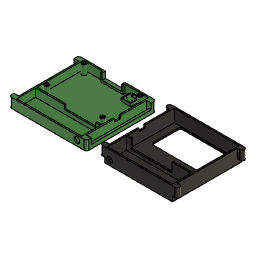
case (Autodesk Fusion 360 design; units mm, degrees)
Autodesk Fusion 360 part; units mm, degrees
(part 1 of 2)
sketch "Sketch1" plane through (0, 0, 0) normal (0, 0, 1) x (1, 0, 0)
  line L0 (0, 0) -> (127, 0)
  line L1 (127, 0) -> (127, 88)
  line L2 (127, 88) -> (0, 88)
  line L3 (0, 88) -> (0, 0)
  circle A0 centre (5, 82.8) radius 3
  circle A1 centre (121.74, 82.8) radius 3
  circle A2 centre (5, 5) radius 3
  circle A3 centre (121.74, 5) radius 3
  circle A4 centre (5, 71.19) radius 3.5
  circle A5 centre (121.74, 71.19) radius 3.5
  circle A6 centre (5, 33.49) radius 3.5
  circle A7 centre (121.74, 33.49) radius 3.5
  line L4 (8, 84.5321) -> (5, 86.2641)
  line L5 (5, 86.2641) -> (2, 84.5321)
  line L6 (2, 84.5321) -> (2, 81.0679)
  line L7 (2, 81.0679) -> (5, 79.3359)
  line L8 (5, 79.3359) -> (8, 81.0679)
  line L9 (8, 81.0679) -> (8, 84.5321)
  line L10 (123.4721, 79.8) -> (125.2041, 82.8)
  line L11 (125.2041, 82.8) -> (123.4721, 85.8)
  line L12 (123.4721, 85.8) -> (120.0079, 85.8)
  line L13 (120.0079, 85.8) -> (118.2759, 82.8)
  line L14 (118.2759, 82.8) -> (120.0079, 79.8)
  line L15 (120.0079, 79.8) -> (123.4721, 79.8)
  line L16 (123.4721, 2) -> (125.2041, 5)
  line L17 (125.2041, 5) -> (123.4721, 8)
  line L18 (123.4721, 8) -> (120.0079, 8)
  line L19 (120.0079, 8) -> (118.2759, 5)
  line L20 (118.2759, 5) -> (120.0079, 2)
  line L21 (120.0079, 2) -> (123.4721, 2)
  line L22 (8, 6.7321) -> (5, 8.4641)
  line L23 (5, 8.4641) -> (2, 6.7321)
  line L24 (2, 6.7321) -> (2, 3.2679)
  line L25 (2, 3.2679) -> (5, 1.5359)
  line L26 (5, 1.5359) -> (8, 3.2679)
  line L27 (8, 3.2679) -> (8, 6.7321)
  point P0 (5, 82.8)
  point P1 (121.74, 82.8)
  point P2 (121.74, 5)
  point P3 (5, 5)
  dimension "d1" = 127
  dimension "d2" = 88
  dimension "d3" = 6
  dimension "d4" = 6
  dimension "d5" = 6
  dimension "d6" = 6
  dimension "d7" = 5.2
  dimension "d8" = 5
  dimension "d9" = 5
  dimension "d10" = 5.26
  dimension "d11" = 7
  dimension "d12" = 7
  dimension "d13" = 7
  dimension "d14" = 7
  dimension "d15" = 11.61
  dimension "d16" = 28.49
  constraint horizontal L0
  constraint vertical L1
  constraint horizontal L2
  constraint vertical L3
  constraint coincident L0.start L3.end
  constraint vertical P0 P3
  constraint vertical P1 P2
  constraint horizontal P0 P1
  constraint horizontal P3 P2
  constraint vertical A4.centre A6.centre
  constraint vertical A5.centre A7.centre
  constraint horizontal A6.centre A7.centre
  constraint horizontal A4.centre A5.centre
  constraint vertical P0 A4.centre
  constraint vertical P1 A5.centre
  constraint coincident P0 A0.centre
  constraint coincident P1 A1.centre
  constraint coincident P2 A3.centre
  constraint coincident P3 A2.centre
  measures "d1" distance of L1.end L2.end
  measures "d2" distance of L0.end L1.end
  measures "d3" diameter of A0
  measures "d4" diameter of A1
  measures "d5" diameter of A2
  measures "d6" diameter of A3
  measures "d7" distance of L2 P0
  measures "d8" distance of L0 P3
  measures "d9" distance of L3 P0
  measures "d10" distance of L1 P1
  measures "d11" diameter of A4
  measures "d12" diameter of A5
  measures "d13" diameter of A6
  measures "d14" diameter of A7
  measures "d15" distance of P0 A4.centre
  measures "d16" distance of P3 A6.centre
extrude "Extrude1" add sketch "Sketch1" along normal blind 1.25 contours L0 L1 L2 L3 | A0 L8 L9 | A0 L4 L9 | A0 L4 L5 | A0 L7 L8 | A0 L5 L6 | A0 L6 L7 | A1 L10 L11 | A1 L11 L12 | A1 L10 L15 | A1 L12 L13 | A1 L14 L15 | A1 L13 L14 | A2 L26 L27 | A2 L22 L27 | A2 L22 L23 | A2 L25 L26 | A2 L23 L24 | A2 L24 L25 | A3 L16 L17 | A3 L17 L18 | A3 L16 L21 | A3 L18 L19 | A3 L20 L21 | A3 L19 L20 makes body 1
extrude "Extrude1'" add sketch "Sketch1" against normal blind 13 separate body contours A0 | A0 L8 L9 | A0 L4 L9 | A0 L4 L5 | A0 L7 L8 | A0 L5 L6 | A0 L6 L7 | A1 | A1 L10 L11 | A1 L11 L12 | A1 L10 L15 | A1 L12 L13 | A1 L14 L15 | A1 L13 L14 | A2 | A2 L26 L27 | A2 L22 L27 | A2 L22 L23 | A2 L25 L26 | A2 L23 L24 | A2 L24 L25 | A3 | A3 L16 L17 | A3 L17 L18 | A3 L16 L21 | A3 L18 L19 | A3 L20 L21 | A3 L19 L20 makes body 2 at (118.8532, 81.8, -4.3333) makes body 3 at (7, 85.1094, -4.3333) makes body 4 at (122.3174, 8, -4.3333) makes body 5 at (8, 4.4226, -4.3333) in component "Component"
extrude "Extrude1''" add sketch "Sketch1" along normal blind 3.25 separate body contours A0 | A1 | A2 | A3 makes body 6 at (7.7644, 81.6347, 1.0833) makes body 7 at (124.5044, 81.6347, 1.0833) makes body 8 at (7.9851, 4.7013, 1.0833) makes body 9 at (121.2191, 7.9544, 2.1667) in component "Component'"
fillet "Fillet1" radius 1 4 edges at (2.203, 81.7152, 3.25) (118.943, 81.7152, 3.25) (2.203, 3.9152, 3.25) (118.943, 3.9152, 3.25) on bodies 6 7 8 9 in component "Component'"
sketch "Sketch2" plane through (0, 0, 1.25) normal (0, 0, 1) x (-1, 0, 0)
  circle A0 centre (-121.74, -82.8) radius 3
  circle A1 centre (-121.74, -5) radius 3
  circle A2 centre (-5, -71.19) radius 3.5
  circle A3 centre (-121.74, -71.19) radius 3.5
  circle A4 centre (-5, -5) radius 3
  circle A5 centre (-5, -33.49) radius 3.5
  circle A6 centre (-121.74, -33.49) radius 3.5
  circle A7 centre (-5, -82.8) radius 3
  line L0 (0, -88) -> (0, 0)
  line L1 (0, 0) -> (-127, 0)
  line L2 (-127, 0) -> (-127, -88)
  line L3 (-127, -88) -> (0, -88)
  line L4 (-8.5, -73.2107) -> (-5, -75.2315)
  line L5 (-5, -75.2315) -> (-1.5, -73.2107)
  line L6 (-1.5, -73.2107) -> (-1.5, -69.1693)
  line L7 (-1.5, -69.1693) -> (-5, -67.1485)
  line L8 (-5, -67.1485) -> (-8.5, -69.1693)
  line L9 (-8.5, -69.1693) -> (-8.5, -73.2107)
  line L10 (-123.7607, -67.69) -> (-125.7815, -71.19)
  line L11 (-125.7815, -71.19) -> (-123.7607, -74.69)
  line L12 (-123.7607, -74.69) -> (-119.7193, -74.69)
  line L13 (-119.7193, -74.69) -> (-117.6985, -71.19)
  line L14 (-117.6985, -71.19) -> (-119.7193, -67.69)
  line L15 (-119.7193, -67.69) -> (-123.7607, -67.69)
  line L16 (-123.7607, -29.99) -> (-125.7815, -33.49)
  line L17 (-125.7815, -33.49) -> (-123.7607, -36.99)
  line L18 (-123.7607, -36.99) -> (-119.7193, -36.99)
  line L19 (-119.7193, -36.99) -> (-117.6985, -33.49)
  line L20 (-117.6985, -33.49) -> (-119.7193, -29.99)
  line L21 (-119.7193, -29.99) -> (-123.7607, -29.99)
  line L22 (-8.5, -35.5107) -> (-5, -37.5315)
  line L23 (-5, -37.5315) -> (-1.5, -35.5107)
  line L24 (-1.5, -35.5107) -> (-1.5, -31.4693)
  line L25 (-1.5, -31.4693) -> (-5, -29.4485)
  line L26 (-5, -29.4485) -> (-8.5, -31.4693)
  line L27 (-8.5, -31.4693) -> (-8.5, -35.5107)
  point P0 (-5, -71.19)
  point P1 (-121.74, -71.19)
  point P2 (-121.74, -33.49)
  point P3 (-5, -33.49)
  constraint coincident P0 A2.centre
  constraint coincident P1 A3.centre
  constraint coincident P2 A6.centre
  constraint coincident P3 A5.centre
extrude "Extrude2" add sketch "Sketch2" along normal blind 8 separate body contours A2 | A2 L5 L6 | A2 L6 L7 | A2 L7 L8 | A2 L4 L5 | A2 L8 L9 | A2 L4 L9 | A3 | A3 L13 L14 | A3 L14 L15 | A3 L12 L13 | A3 L10 L15 | A3 L11 L12 | A3 L10 L11 | A5 | A5 L23 L24 | A5 L24 L25 | A5 L25 L26 | A5 L22 L23 | A5 L26 L27 | A5 L22 L27 | A6 | A6 L19 L20 | A6 L20 L21 | A6 L18 L19 | A6 L16 L21 | A6 L17 L18 | A6 L16 L17 makes body 10 at (6.1667, 34.1636, 1.25) makes body 11 at (122.4136, 72.3567, 9.25) makes body 12 at (3.8333, 71.8636, 1.25) makes body 13 at (121.0664, 34.6567, 9.25)
sketch "Sketch3" plane through (0, 0, 9.25) normal (0, 0, 1) x (-1, 0, 0)
  line L0 (-8.5, -69.1693) -> (-8.5, -73.2107)
  line L1 (-8.5, -73.2107) -> (-5, -75.2315)
  line L2 (-5, -75.2315) -> (-1.5, -73.2107)
  line L3 (-1.5, -73.2107) -> (-1.5, -69.1693)
  line L4 (-1.5, -69.1693) -> (-5, -67.1485)
  line L5 (-5, -67.1485) -> (-8.5, -69.1693)
  line L6 (0, -88) -> (-127, -88)
  line L7 (-127, -88) -> (-127, -28)
  line L8 (-127, -28) -> (0, -28)
  line L9 (0, -28) -> (0, -88)
  dimension "d27" = 127
  dimension "d28" = 60
  dimension "d29" = 88
  constraint horizontal L6
  constraint vertical L7
  constraint horizontal L8
  constraint vertical L9
  constraint collinear origin L6.start L8.end
  measures "d27" distance of L6.start L6.end
  measures "d28" distance of L6.start L8.end
  measures "d29" vertical distance of origin L6.start
extrude "Extrude1'''" add sketch "Sketch3" along normal blind 1.65 separate body contours L0 L1 L2 L3 L4 L5 | L6 L7 L8 L9 makes body 14 in component "Component''"
sketch "Sketch4" plane through (0, 0, 10.9) normal (0, 0, 1) x (-1, 0, 0)
  line L0 (0, -28) -> (-127, -28)
  line L1 (-127, -28) -> (-127, -88)
  line L2 (-127, -88) -> (0, -88)
  line L3 (0, -88) -> (0, -28)
  circle A0 centre (-5, -71.19) radius 3.5
  circle A1 centre (-5, -33.49) radius 3.5
  circle A2 centre (-121.74, -71.19) radius 3.5
  circle A3 centre (-121.74, -33.49) radius 3.5
  circle A4 centre (-5, -71.19) radius 3.5
  circle A5 centre (-5, -33.49) radius 3.5
  circle A6 centre (-121.74, -71.19) radius 3.5
  circle A7 centre (-121.74, -33.49) radius 3.5
  line L4 (-14, -88) -> (-113, -88)
  line L5 (-117, -84) -> (-117, -32)
  line L6 (-113, -28) -> (-14, -28)
  line L7 (-10, -32) -> (-10, -84)
  line L8 (-127, -88) -> (0, -88)
  line L9 (-127, 0) -> (-127, -88)
  arc A8 (-14, -88) -> (-10, -84) centre (-14, -84) ccw
  arc A9 (-10, -32) -> (-14, -28) centre (-14, -32) ccw
  arc A10 (-113, -28) -> (-117, -32) centre (-113, -32) ccw
  arc A11 (-117, -84) -> (-113, -88) centre (-113, -84) ccw
  dimension "d33" = 7
  dimension "d34" = 7
  dimension "d35" = 7
  dimension "d36" = 7
  dimension "d37" = 107
  dimension "d38" = 10
  dimension "d39" = 4
  dimension "d40" = 4
  constraint concentric A0 A4
  constraint concentric A1 A5
  constraint concentric A2 A6
  constraint concentric A3 A7
  constraint horizontal L4
  constraint vertical L5
  constraint horizontal L6
  constraint vertical L7
  constraint collinear L4 L8
  constraint collinear L0 L6
  constraint tangent L4 A8
  constraint tangent L7 A8
  constraint tangent L6 A9
  constraint tangent L7 A9
  constraint tangent L5 A10
  constraint tangent L6 A10
  constraint equal A9 A10
  constraint tangent L4 A11
  constraint tangent L5 A11
  constraint equal A9 A11
  measures "d33" diameter of A0
  measures "d34" diameter of A1
  measures "d35" diameter of A2
  measures "d36" diameter of A3
  measures "d37" distance of L5 L7
  measures "d38" distance of L5 L9
  measures "d39" radius of A8
  measures "d40" radius of A9
extrude "Extrude1''''" add sketch "Sketch4" along normal blind 2 separate body contours A0 A4 | A1 A5 | A2 A6 | A3 A7 makes body 15 at (124.0559, 36.1142, 12.2333) makes body 16 at (1.5174, 33.8385, 11.5667) makes body 17 at (124.0559, 73.8142, 12.2333) makes body 18 at (1.7748, 72.5495, 11.5667) in component "Component'''"
extrude "Extrude1'''''" add sketch "Sketch4" along normal blind 3 separate body contours L0 L2 L4 L5 L6 L7 L8 A8 A9 A10 A11 makes body 19 in component "Component''''"
fillet "Fillet1'" radius 1 4 edges at (125.0031, 34.7557, 12.9) (8.2631, 34.7557, 12.9) (125.0031, 72.4557, 12.9) (8.2631, 72.4557, 12.9) on bodies 15 16 17 18 in component "Component'''"
extrude "Extrude1''''''" add sketch "Sketch1" against normal blind 2 separate body contours A4 | A5 | A6 | A7 makes body 20 at (120.6253, 30.1723, -1.3333) makes body 21 at (8.4956, 33.3155, -1.3333) makes body 22 at (119.2962, 68.6845, -1.3333) makes body 23 at (8.2889, 69.9929, -1.3333) in component "Component'''''"
fillet "Fillet1''" radius 1 4 edges at (118.4769, 34.7557, -2) (1.7369, 34.7557, -2) (118.4769, 72.4557, -2) (1.7369, 72.4557, -2) on bodies 20 21 22 23 in component "Component'''''"
sketch "Sketch5" plane through (0, 0, 0) normal (0, 0, -1) x (1, 0, 0)
  circle A0 centre (121.74, -82.8) radius 3
  circle A1 centre (121.74, -5) radius 3
  circle A2 centre (5, -71.19) radius 3.5
  circle A3 centre (121.74, -71.19) radius 3.5
  circle A4 centre (5, -5) radius 3
  circle A5 centre (5, -33.49) radius 3.5
  circle A6 centre (121.74, -33.49) radius 3.5
  circle A7 centre (5, -82.8) radius 3
  line L0 (0, 0) -> (0, -88)
  line L1 (0, -88) -> (127, -88)
  line L2 (127, -88) -> (127, 0)
  line L3 (127, 0) -> (0, 0)
  line L4 (75.75, -5.5) -> (83.75, -5.5)
  line L5 (83.75, -5.5) -> (83.75, 0)
  line L6 (83.75, 0) -> (75.75, 0)
  line L7 (75.75, 0) -> (75.75, -5.5)
  line L8 (90.75, -5.5) -> (98.75, -5.5)
  line L9 (98.75, -5.5) -> (98.75, 0)
  line L10 (98.75, 0) -> (90.75, 0)
  line L11 (90.75, 0) -> (90.75, -5.5)
  line L12 (35, -20.5) -> (37.5, -20.5)
  line L13 (37.5, -20.5) -> (37.5, -68.5)
  line L14 (37.5, -68.5) -> (35, -68.5)
  line L15 (35, -68.5) -> (35, -20.5)
  line L16 (83, -20.5) -> (85.5, -20.5)
  line L17 (85.5, -20.5) -> (85.5, -59)
  line L18 (85.5, -59) -> (83, -59)
  line L19 (83, -59) -> (83, -20.5)
  line L20 (114.7, -42) -> (130, -42)
  line L21 (130, -42) -> (130, -58.25)
  line L22 (130, -58.25) -> (114.7, -58.25)
  line L23 (114.7, -58.25) -> (114.7, -42)
  line L24 (21, -71.95) -> (27, -71.95)
  line L25 (27, -71.95) -> (27, -89.25)
  line L26 (27, -89.25) -> (21, -89.25)
  line L27 (21, -89.25) -> (21, -71.95)
  line L28 (38.2, -71.95) -> (44.2, -71.95)
  line L29 (44.2, -71.95) -> (44.2, -89.25)
  line L30 (44.2, -89.25) -> (38.2, -89.25)
  line L31 (38.2, -89.25) -> (38.2, -71.95)
  line L32 (15.5, -66.5) -> (-0.5, -66.5)
  line L33 (-0.5, -66.5) -> (-0.5, -55.5)
  line L34 (-0.5, -55.5) -> (15.5, -55.5)
  line L35 (15.5, -55.5) -> (15.5, -66.5)
  line L36 (15.5, -49) -> (-0.5, -49)
  line L37 (-0.5, -49) -> (-0.5, -38)
  line L38 (-0.5, -38) -> (15.5, -38)
  line L39 (15.5, -38) -> (15.5, -49)
  line L40 (75.75, 0) -> (83.75, 0)
  line L41 (83.75, 0) -> (83.75, 1.25)
  line L42 (83.75, 1.25) -> (75.75, 1.25)
  line L43 (75.75, 1.25) -> (75.75, 0)
  line L44 (90.75, 0) -> (98.75, 0)
  line L45 (98.75, 0) -> (98.75, 1.25)
  line L46 (98.75, 1.25) -> (90.75, 1.25)
  line L47 (90.75, 1.25) -> (90.75, 0)
  dimension "d51" = 8
  dimension "d52" = 8
  dimension "d53" = 5.5
  dimension "d54" = 5.5
  dimension "d55" = 36.25
  dimension "d56" = 23
  dimension "d57" = 16.25
  dimension "d58" = 15.3
  dimension "d59" = 3
  dimension "d60" = 46
  dimension "d61" = 6
  dimension "d62" = 6
  dimension "d63" = 17.3
  dimension "d64" = 17.3
  dimension "d65" = 1.25
  dimension "d66" = 1.25
  dimension "d67" = 27
  dimension "d68" = 23.2
  dimension "d69" = 11
  dimension "d70" = 11
  dimension "d71" = 16
  dimension "d72" = 16
  dimension "d73" = 0.5
  dimension "d74" = 0.5
  dimension "d75" = 50
  dimension "d76" = 28.5
  dimension "d77" = 48
  dimension "d78" = 38.5
  dimension "d79" = 2.5
  dimension "d80" = 2.5
  dimension "d81" = 20.5
  dimension "d82" = 67.5
  dimension "d83" = 44
  dimension "d84" = 50.5
  dimension "d122" = 1.25
  constraint horizontal L4
  constraint vertical L5
  constraint horizontal L6
  constraint vertical L7
  constraint coincident L3 L5.end
  constraint horizontal L8
  constraint vertical L9
  constraint horizontal L10
  constraint vertical L11
  constraint coincident L3 L9.end
  constraint horizontal L12
  constraint vertical L13
  constraint horizontal L14
  constraint vertical L15
  constraint horizontal L16
  constraint vertical L17
  constraint horizontal L18
  constraint vertical L19
  constraint horizontal L20
  constraint vertical L21
  constraint horizontal L22
  constraint vertical L23
  constraint horizontal L24
  constraint vertical L25
  constraint horizontal L26
  constraint vertical L27
  constraint horizontal L28
  constraint vertical L29
  constraint horizontal L30
  constraint vertical L31
  constraint horizontal L32
  constraint vertical L33
  constraint horizontal L34
  constraint vertical L35
  constraint horizontal L36
  constraint vertical L37
  constraint horizontal L38
  constraint vertical L39
  constraint horizontal L40
  constraint vertical L41
  constraint horizontal L42
  constraint vertical L43
  constraint horizontal L44
  constraint vertical L45
  constraint horizontal L46
  constraint vertical L47
  constraint collinear L42 L46
  measures "d51" distance of L4.start L4.end
  measures "d52" distance of L8.start L8.end
  measures "d53" distance of L4.end L5.end
  measures "d54" distance of L8.start L10.end
  measures "d55" distance of L2 L11
  measures "d56" distance of L7 L9
  measures "d57" distance of L20.end L21.end
  measures "d58" distance of L20.start L20.end
  measures "d59" distance of L2 L21
  measures "d60" vertical distance of L1.end L20.end
  measures "d61" distance of L25.end L26.end
  measures "d62" distance of L29.end L30.end
  measures "d63" distance of L24.start L26.end
  measures "d64" distance of L28.end L29.end
  measures "d65" distance of L1 L25.end
  measures "d66" distance of L1 L30.end
  measures "d67" horizontal distance of L0.end L25.end
  measures "d68" distance of L27 L29
  measures "d69" distance of L36.end L37.end
  measures "d70" distance of L32.end L33.end
  measures "d71" distance of L32.start L32.end
  measures "d72" distance of L37.end L38.end
  measures "d73" distance of L0 L37.end
  measures "d74" distance of L0 L32.end
  measures "d75" distance of L1 L38
  measures "d76" distance of L32 L38
  measures "d77" distance of L12.end L13.end
  measures "d78" distance of L16.end L17.end
  measures "d79" distance of L12.start L12.end
  measures "d80" distance of L16.start L16.end
  measures "d81" distance of L3 L12.end
  measures "d82" distance of L1 L16.start
  measures "d83" distance of L2 L19
  measures "d84" distance of L15 L17
  measures "d122" distance of L6.end L42.end
extrude "Extrude1'''''''" add sketch "Sketch5" along normal blind 5 separate body contours L1 L24 L25 L27 | L1 L25 L26 L27 | L1 L28 L29 L31 | L1 L29 L30 L31 makes body 24 at (23, 83.4833, 0) makes body 25 at (40.2, 77.7167, 0) in component "Component''''''"
extrude "Extrude1''''''''" add sketch "Sketch5" along normal blind 7 and the other way blind 5 separate body contours L2 L20 L21 L22 | L2 L20 L22 L23 makes body 26 in component "Component'''''''"
extrude "Extrude1'''''''''" add sketch "Sketch5" along normal blind 3 separate body contours L3 L6 L40 L41 L42 L43 | L3 L4 L5 L6 L7 L40 | L3 L10 L44 L45 L46 L47 | L3 L8 L9 L10 L11 L44 makes body 27 at (78.4167, 1, 0) makes body 28 at (93.4167, 1, 0) in component "Component''''''''"
extrude "Extrude1''''''''''" add sketch "Sketch5" along normal blind 12 separate body contours L0 L36 L38 L39 | L0 L36 L37 L38 | L0 L32 L34 L35 | L0 L32 L33 L34 makes body 29 at (4.8333, 38, -4) makes body 30 at (4.8333, 55.5, -4) in component "Component'''''''''"
extrude "Extrude3" add sketch "Sketch5" along normal blind 11 contours L12 L13 L14 L15 | L16 L17 L18 L19 bodies 1
sketch "Sketch6" plane through (0, 0, -11) normal (0, 0, -1) x (1, 0, 0)
  line L0 (35, -68.5) -> (37.5, -68.5)
  line L1 (37.5, -68.5) -> (37.5, -20.5)
  line L2 (37.5, -20.5) -> (35, -20.5)
  line L3 (35, -20.5) -> (35, -68.5)
  line L4 (33, -14.5) -> (98, -14.5)
  line L5 (98, -14.5) -> (98, -88)
  line L6 (98, -88) -> (33, -88)
  line L7 (33, -88) -> (33, -14.5)
  point P0 (0, -88)
  dimension "d97" = 73.5
  dimension "d98" = 65
  dimension "d103" = 88
  dimension "d104" = 98
  constraint horizontal L4
  constraint vertical L5
  constraint horizontal L6
  constraint vertical L7
  measures "d97" distance of L4 L6
  measures "d98" distance of L4.start L4.end
  measures "d103" distance of origin L6
  measures "d104" distance of L5.end P0
extrude "Extrude1'''''''''''" add sketch "Sketch6" along normal blind 1.65 separate body contours L0 L1 L2 L3 | L4 L5 L6 L7 makes body 31 in component "Component''''''''''"
sketch "Sketch7" plane through (0, 0, -12.65) normal (0, 0, -1) x (1, 0, 0)
  line L0 (33, -88) -> (98, -88)
  line L1 (98, -88) -> (98, -14.5)
  line L2 (98, -14.5) -> (33, -14.5)
  line L3 (33, -14.5) -> (33, -88)
  line L4 (40, -73) -> (79.25, -73)
  line L5 (79.25, -73) -> (79.25, -88)
  line L6 (79.25, -88) -> (40, -88)
  line L7 (40, -88) -> (40, -73)
  point P0 (0, -88)
  dimension "d105" = 39.25
  dimension "d106" = 15
  dimension "d107" = 7
  constraint horizontal L4
  constraint vertical L5
  constraint horizontal L6
  constraint vertical L7
  constraint collinear L5.end L6.end P0
  measures "d105" distance of L5.end L6.end
  measures "d106" distance of L4.end L5.end
  measures "d107" distance of L3 L7
extrude "Extrude1''''''''''''" add sketch "Sketch7" along normal blind 12.5 separate body contours L0 L4 L5 L6 L7 makes body 32 in component "Component'''''''''''"
sketch "Sketch8" plane through (0, 88, 0) normal (0, 1, 0) x (-1, 0, 0)
  line L0 (-40, -12.65) -> (-79.25, -12.65)
  line L1 (-79.25, -12.65) -> (-79.25, -25.15)
  line L2 (-79.25, -25.15) -> (-40, -25.15)
  line L3 (-40, -25.15) -> (-40, -12.65)
  line L4 (-72.125, -14.9) -> (-47.125, -14.9)
  line L5 (-47.125, -14.9) -> (-47.125, -22.9)
  line L6 (-47.125, -22.9) -> (-72.125, -22.9)
  line L7 (-72.125, -22.9) -> (-72.125, -14.9)
  circle A0 centre (-76.25, -19.15) radius 2.5
  circle A1 centre (-43, -19.15) radius 2.5
  dimension "d110" = 8
  dimension "d111" = 25
  dimension "d112" = 5
  dimension "d113" = 5
  dimension "d114" = 6.5
  dimension "d116" = 2.25
  dimension "d117" = 7.125
  dimension "d118" = 3
  dimension "d119" = 3
  constraint horizontal L4
  constraint vertical L5
  constraint horizontal L6
  constraint vertical L7
  constraint horizontal A0.centre A1.centre
  measures "d110" distance of L4.end L5.end
  measures "d111" distance of L4.start L4.end
  measures "d112" diameter of A0
  measures "d113" diameter of A1
  measures "d114" distance of L0 A0.centre
  measures "d116" distance of L2 L6
  measures "d117" distance of L3 L5
  measures "d118" distance of L1 A0.centre
  measures "d119" distance of L3 A1.centre
extrude "Extrude2'" add sketch "Sketch8" along normal blind 6 contours L4 L5 L6 L7 | A0 | A1 bodies 32 in component "Component'''''''''''"
sketch "Sketch9" plane through (0, 0, 0) normal (0, 0, 1) x (1, 0, 0)
  line L0 (-145.3464, 58.1125) -> (-35.3464, 58.1125)
  line L1 (-35.3464, 58.1125) -> (-35.3464, 23.1125)
  line L2 (-35.3464, 23.1125) -> (-145.3464, 23.1125)
  line L3 (-145.3464, 23.1125) -> (-145.3464, 58.1125)
  dimension "d123" = 35
  dimension "d124" = 110
  constraint horizontal L0
  constraint vertical L1
  constraint horizontal L2
  constraint vertical L3
  measures "d123" distance of L0 L2
  measures "d124" distance of L0.start L0.end
extrude "Extrude4" add sketch "Sketch9" along normal blind 30 separate body makes body 33
move_body "Move1" bodies 33 to x (1, 0, 0) y (0, 1, 0) z (0, 0, 1) at (0, 0, -25)
move_body "Move2" bodies 33 to x (1, 0, 0) y (0, 1, 0) z (0, 0, 1) at (155, -70, 0)
move_body "Move3" bodies 33 to x (1, 0, 0) y (0, 1, 0) z (0, 0, 1) at (0, 0, 5)
move_body "Move4" bodies 33 to x (1, 0, 0) y (0, 1, 0) z (0, 0, 1) at (0, 0, -5)
move_body "Move5" bodies 33 to x (1, 0, 0) y (0, 1, 0) z (0, 0, 1) at (-10, 0, 0)
move_body "Move6" bodies 33 to x (1, 0, 0) y (0, 1, 0) z (0, 0, 1) at (2, 0, 0)
sketch "Sketch10" plane through (0, 0, 0) normal (0, 0, 1) x (1, 0, 0)
  line L0 (-6, 93) -> (135, 93)
  line L1 (135, 93) -> (135, -52)
  line L2 (135, -52) -> (-6, -52)
  line L3 (-6, -52) -> (-6, 93)
  line L4 (132, -49) -> (-3, -49)
  line L5 (-3, -49) -> (-3, 90)
  line L6 (-3, 90) -> (132, 90)
  line L7 (132, 90) -> (132, -49)
  line L8 (-3, -7) -> (132, -7)
  line L9 (-3, -10) -> (132, -10)
  dimension "d127" = 6
  dimension "d128" = 141
  dimension "d129" = 145
  dimension "d130" = 93
  dimension "d131" = 3
  dimension "d132" = 3
  dimension "d133" = 39
  constraint horizontal L0
  constraint vertical L1
  constraint horizontal L2
  constraint vertical L3
  constraint coincident L5 L8.start
  constraint coincident L7 L8.end
  constraint perpendicular L7 L8
  constraint coincident L5 L9.start
  constraint coincident L7 L9.end
  constraint perpendicular L7 L9
  measures "d127" distance of origin L3
  measures "d128" distance of L1 L3
  measures "d129" distance of L0 L2
  measures "d130" vertical distance of origin L0.start
  measures "d132" distance of L8 L9
  measures "d133" distance of L4 L9
move_body "Move7" bodies 33 to x (1, 0, 0) y (0, 1, 0) z (0, 0, 1) at (0, -2, 0)
move_body "Move8" bodies 33 to x (1, 0, 0) y (0, 1, 0) z (0, 0, 1) at (-2, 0, 0)
move_body "Move1'" bodies 25 24 to x (1, 0, 0) y (0, 1, 0) z (0, 0, 1) at (150, 0, 0) in component "Component''''''"
move_body "Move1''" bodies 26 to x (1, 0, 0) y (0, 1, 0) z (0, 0, 1) at (150, 0, 0) in component "Component'''''''"
move_body "Move9" bodies 10 33 12 1 11 13 to x (1, 0, 0) y (0, 1, 0) z (0, 0, 1) at (150, 0, 0)
move_body "Move1'''" bodies 18 17 16 15 to x (1, 0, 0) y (0, 1, 0) z (0, 0, 1) at (150, 0, 0) in component "Component'''"
move_body "Move1''''" bodies 21 22 23 20 to x (1, 0, 0) y (0, 1, 0) z (0, 0, 1) at (150, 0, 0) in component "Component'''''"
move_body "Move1'''''" bodies 5 2 3 4 to x (1, 0, 0) y (0, 1, 0) z (0, 0, 1) at (150, 0, 0) in component "Component"
move_body "Move1''''''" bodies 19 to x (1, 0, 0) y (0, 1, 0) z (0, 0, 1) at (150, 0, 0) in component "Component''''"
move_body "Move1'''''''" bodies 14 to x (1, 0, 0) y (0, 1, 0) z (0, 0, 1) at (150, 0, 0) in component "Component''"
move_body "Move1''''''''" bodies 6 8 9 7 to x (1, 0, 0) y (0, 1, 0) z (0, 0, 1) at (150, 0, 0) in component "Component'"
move_body "Move1'''''''''" bodies 31 to x (1, 0, 0) y (0, 1, 0) z (0, 0, 1) at (150, 0, 0) in component "Component''''''''''"
move_body "Move1''''''''''" bodies 32 to x (1, 0, 0) y (0, 1, 0) z (0, 0, 1) at (150, 0, 0) in component "Component'''''''''''"
move_body "Move1'''''''''''" bodies 29 30 to x (1, 0, 0) y (0, 1, 0) z (0, 0, 1) at (150, 0, 0) in component "Component'''''''''"
move_body "Move1''''''''''''" bodies 27 28 to x (1, 0, 0) y (0, 1, 0) z (0, 0, 1) at (150, 0, 0) in component "Component''''''''"
extrude "Extrude5" add sketch "Sketch10" against normal blind 17 separate body contours L0 L1 L2 L3 | L5 L7 L8 L9 makes body 34
sketch "Sketch11" plane through (0, 0, -17) normal (0, 0, -1) x (1, 0, 0)
  line L0 (-3, -90) -> (-3, 7)
  line L1 (-3, 7) -> (132, 7)
  line L2 (132, 7) -> (132, -90)
  line L3 (132, -90) -> (-3, -90)
  line L4 (-3, 10) -> (-3, 49)
  line L5 (-3, 49) -> (132, 49)
  line L6 (132, 49) -> (132, 10)
  line L7 (132, 10) -> (-3, 10)
  line L8 (135, 52) -> (-6, 52)
  line L9 (-6, 52) -> (-6, -93)
  line L10 (-6, -93) -> (135, -93)
  line L11 (135, -93) -> (135, 52)
  line L12 (-6, 52) -> (135, 52)
  line L13 (135, 52) -> (135, -93)
  line L14 (135, -93) -> (-6, -93)
  line L15 (-6, -93) -> (-6, 52)
  dimension "d136" = 145
  dimension "d137" = 141
  constraint horizontal L12
  constraint vertical L13
  constraint horizontal L14
  constraint vertical L15
  constraint coincident L8.end L9.start
  measures "d136" distance of L8.start L10.end
  measures "d137" distance of L10.end L9.end
extrude "Extrude6" add sketch "Sketch11" along normal blind 3 contours L0 L1 L2 L3 | L4 L5 L6 L7 | L8 L9 L10 L11 L12 L13 L14 L15 bodies 34
move_body "Move10" bodies 34 to x (1, 0, 0) y (0, 1, 0) z (0, 0, 1) at (0, 0, -12.65)
move_body "Move11" bodies 34 to x (1, 0, 0) y (0, 1, 0) z (0, 0, 1) at (150, 0, 0)
sketch "Sketch12" plane through (0, 93, 0) normal (0, 1, 0) x (-1, 0, 0)
  line L0 (-144, -12.65) -> (-285, -12.65)
  line L1 (-285, -12.65) -> (-285, -32.65)
  line L2 (-285, -32.65) -> (-144, -32.65)
  line L3 (-144, -32.65) -> (-144, -12.65)
  line L4 (-230, -12.65) -> (-189.5, -12.65)
  line L5 (-189.5, -12.65) -> (-189.5, -25.65)
  line L6 (-189.5, -25.65) -> (-230, -25.65)
  line L7 (-230, -25.65) -> (-230, -12.65)
  line L8 (-233, -12.65) -> (-233, -32.65)
  line L9 (-186.5, -32.65) -> (-186.5, -12.65)
  dimension "d140" = 40.5
  dimension "d141" = 13
  dimension "d142" = 55
  dimension "d149" = 3
  dimension "d150" = 3
  constraint horizontal L4
  constraint vertical L5
  constraint horizontal L6
  constraint vertical L7
  constraint collinear L0 L4
  constraint coincident L0 L8.start
  constraint coincident L2 L8.end
  constraint perpendicular L2 L8
  constraint coincident L2 L9.start
  constraint coincident L0 L9.end
  constraint perpendicular L0 L9
  measures "d140" distance of L5.end L6.end
  measures "d141" distance of L4.end L5.end
  measures "d142" distance of L1 L7
  measures "d149" distance of L7 L8
  measures "d150" distance of L5 L9
extrude "Extrude7" cut sketch "Sketch12" against normal blind 3 contours L0 L4 L5 L6 L7 bodies 34
extrude "Extrude8" add sketch "Sketch12" against normal blind 7 contours L0 L2 L5 L6 L7 L8 L9 bodies 34
extrude "Extrude9" add sketch "Sketch11" against normal blind 26 separate body makes body 35
extrude "Extrude10" add sketch "Sketch11" against normal blind 3 from surface at -26 contours L0 L1 L2 L3 | L4 L5 L6 L7 | L8 L9 L10 L11 L12 L13 L14 L15 bodies 35
move_body "Move12" bodies 35 to x (1, 0, 0) y (0, 1, 0) z (0, 0, 1) at (0, 0, 4.35)
move_body "Move13" bodies 35 to x (1, 0, 0) y (0, 1, 0) z (0, 0, 1) at (150, 0, 0)
sketch "Sketch13" plane through (0, 0, 16.35) normal (0, 0, 1) x (-1, 0, 0)
  line L0 (-285, -93) -> (-144, -93)
  line L1 (-144, -93) -> (-144, 52)
  line L2 (-144, 52) -> (-285, 52)
  line L3 (-285, 52) -> (-285, -93)
  line L4 (-164, -88.5) -> (-263, -88.5)
  line L5 (-268, -83.5) -> (-268, -32.5)
  line L6 (-263, -27.5) -> (-164, -27.5)
  line L7 (-159, -32.5) -> (-159, -83.5)
  arc A0 (-164, -88.5) -> (-159, -83.5) centre (-164, -83.5) ccw
  arc A1 (-159, -32.5) -> (-164, -27.5) centre (-164, -32.5) ccw
  arc A2 (-263, -27.5) -> (-268, -32.5) centre (-263, -32.5) ccw
  arc A3 (-268, -83.5) -> (-263, -88.5) centre (-263, -83.5) ccw
  dimension "d158" = 4.5
  dimension "d159" = 15
  dimension "d160" = 17
  dimension "d161" = 61
  dimension "d162" = 5
  constraint horizontal L4
  constraint vertical L5
  constraint horizontal L6
  constraint vertical L7
  constraint tangent L4 A0
  constraint tangent L7 A0
  constraint tangent L6 A1
  constraint tangent L7 A1
  constraint equal A0 A1
  constraint tangent L5 A2
  constraint tangent L6 A2
  constraint equal A0 A2
  constraint tangent L4 A3
  constraint tangent L5 A3
  constraint equal A0 A3
  measures "d158" distance of L0 L4
  measures "d159" distance of L1 L7
  measures "d160" distance of L3 L5
  measures "d161" distance of L4 L6
  measures "d162" radius of A0
extrude "Extrude11" cut sketch "Sketch13" against normal blind 3 contours L4 L5 L6 L7 A0 A1 A2 A3 bodies 35
extrude "Extrude2''" cut sketch "Sketch13" against normal blind 3 contours L4 L5 L6 L7 A0 A1 A2 A3 bodies 19 in component "Component''''"
move_body "Move14" bodies 35 to x (1, 0, 0) y (0, 1, 0) z (0, 0, 1) at (-170, 0, 0)
move_body "Move15" bodies 33 to x (1, 0, 0) y (0, 1, 0) z (0, 0, 1) at (0, 2, 0)
sketch "Sketch15" plane through (0, 0, -29.65) normal (0, 0, 1) x (-1, 0, 0)
  line L0 (-186.5, -86) -> (-186.5, -90)
  line L1 (-186.5, -90) -> (-147, -90)
  line L2 (-147, -90) -> (-147, 7)
  line L3 (-147, 7) -> (-282, 7)
  line L4 (-282, 7) -> (-282, -90)
  line L5 (-282, -90) -> (-233, -90)
  line L6 (-233, -90) -> (-233, -86)
  line L7 (-233, -86) -> (-186.5, -86)
  circle A0 centre (-155, -82.8) radius 4.5
  circle A1 centre (-155, -5) radius 4.5
  circle A2 centre (-271.74, -82.8) radius 4.5
  circle A3 centre (-271.74, -5) radius 4.5
  circle A4 centre (-155, -71.19) radius 3.5
  circle A5 centre (-271.74, -71.19) radius 2.5
  circle A6 centre (-271.74, -33.49) radius 2.5
  circle A7 centre (-155, -33.49) radius 2.5
  circle A8 centre (-155, -82.8) radius 3
  circle A9 centre (-155, -5) radius 3
  circle A10 centre (-271.74, -82.8) radius 3
  circle A11 centre (-271.74, -5) radius 3
  dimension "d167" = 9
  dimension "d168" = 9
  dimension "d169" = 9
  dimension "d170" = 9
  constraint concentric A0 A8
  constraint concentric A1 A9
  constraint concentric A2 A10
  constraint concentric A3 A11
  measures "d167" diameter of A0
  measures "d168" diameter of A1
  measures "d169" diameter of A2
  measures "d170" diameter of A3
extrude "Extrude12" add sketch "Sketch15" along normal blind 16.65 contours A0 | A1 | A2 | A3 | A8 | A9 | A10 | A11 bodies 34
sketch "Sketch16" plane through (0, 0, -13) normal (0, 0, 1) x (-1, 0, 0)
  circle A0 centre (-155, -82.8) radius 4.5
  line L0 (-158, -84.5321) -> (-155, -86.2641)
  line L1 (-155, -86.2641) -> (-152, -84.5321)
  line L2 (-152, -84.5321) -> (-152, -81.0679)
  line L3 (-152, -81.0679) -> (-155, -79.3359)
  line L4 (-155, -79.3359) -> (-158, -81.0679)
  line L5 (-158, -81.0679) -> (-158, -84.5321)
  line L6 (-271.74, -86.2641) -> (-268.74, -84.5321)
  line L7 (-271.74, -79.3359) -> (-274.74, -81.0679)
  line L8 (-274.74, -84.5321) -> (-271.74, -86.2641)
  line L9 (-274.74, -81.0679) -> (-274.74, -84.5321)
  line L10 (-268.74, -84.5321) -> (-268.74, -81.0679)
  line L11 (-268.74, -81.0679) -> (-271.74, -79.3359)
  line L12 (-155, -8.4641) -> (-152, -6.7321)
  line L13 (-155, -1.5359) -> (-158, -3.2679)
  line L14 (-158, -6.7321) -> (-155, -8.4641)
  line L15 (-158, -3.2679) -> (-158, -6.7321)
  line L16 (-152, -6.7321) -> (-152, -3.2679)
  line L17 (-152, -3.2679) -> (-155, -1.5359)
  line L18 (-271.74, -8.4641) -> (-268.74, -6.7321)
  line L19 (-271.74, -1.5359) -> (-274.74, -3.2679)
  line L20 (-274.74, -6.7321) -> (-271.74, -8.4641)
  line L21 (-274.74, -3.2679) -> (-274.74, -6.7321)
  line L22 (-268.74, -6.7321) -> (-268.74, -3.2679)
  line L23 (-268.74, -3.2679) -> (-271.74, -1.5359)
  circle A1 centre (-155, -5) radius 4.5
  circle A2 centre (-271.74, -5) radius 4.5
  circle A3 centre (-271.74, -82.8) radius 4.5
  point P0 (-155, -82.8)
  point P1 (-271.74, -82.8)
  point P2 (-271.74, -82.8)
  point P3 (-155, -5)
  point P4 (-155, -5)
  point P5 (-271.74, -5)
  point P6 (-271.74, -5)
  dimension "d173" = 3
  dimension "d176" = -116.74
  dimension "d177" = 77.8
  dimension "d178" = 9
  dimension "d179" = 9
  dimension "d180" = 9
  constraint coincident P0 A0.centre
  constraint vertical L5
  constraint coincident P4 P3
  constraint coincident P6 P5
  constraint coincident P2 P1
  measures "d173" distance of P0 L5
  measures "d178" diameter of A1
  measures "d179" diameter of A2
  measures "d180" diameter of A3
extrude "Extrude13" add sketch "Sketch16" along normal blind 3 bodies 34
move_body "Move2'" bodies 2 to x (0.866025, -0.5, 0) y (0.5, 0.866025, 0) z (0, 0, 1) at (-4.9937, 146.9631, 0) in component "Component"
move_body "Move3'" bodies 4 to x (0.866025, -0.5, 0) y (0.5, 0.866025, 0) z (0, 0, 1) at (33.9063, 136.5399, 0) in component "Component"
sketch "Sketch17" plane through (0, 0, 16.35) normal (0, 0, 1) x (-1, 0, 0)
  line L0 (-98, -83.5) -> (-98, -32.5)
  arc A0 (-93, -27.5) -> (-98, -32.5) centre (-93, -32.5) ccw
  line L1 (-93, -27.5) -> (6, -27.5)
  arc A1 (11, -32.5) -> (6, -27.5) centre (6, -32.5) ccw
  line L2 (11, -32.5) -> (11, -83.5)
  arc A2 (6, -88.5) -> (11, -83.5) centre (6, -83.5) ccw
  line L3 (6, -88.5) -> (-93, -88.5)
  arc A3 (-98, -83.5) -> (-93, -88.5) centre (-93, -83.5) ccw
  line L4 (-115, -93) -> (26, -93)
  line L5 (26, -93) -> (26, 52)
  line L6 (26, 52) -> (-115, 52)
  line L7 (-115, 52) -> (-115, -93)
  line L8 (26, -93) -> (36, -93)
  line L9 (36, -93) -> (36, -83)
  line L10 (36, -83) -> (26, -83)
  line L11 (26, -83) -> (26, -93)
  line L12 (26, 52) -> (36, 52)
  line L13 (36, 52) -> (36, 42)
  line L14 (36, 42) -> (26, 42)
  line L15 (26, 42) -> (26, 52)
  line L16 (-115, 52) -> (-125, 52)
  line L17 (-125, 52) -> (-125, 42)
  line L18 (-125, 42) -> (-115, 42)
  line L19 (-115, 42) -> (-115, 52)
  line L20 (-115, -93) -> (-125, -93)
  line L21 (-125, -93) -> (-125, -83)
  line L22 (-125, -83) -> (-115, -83)
  line L23 (-115, -83) -> (-115, -93)
  dimension "d185" = 10
  dimension "d186" = 10
  dimension "d187" = 10
  dimension "d188" = 10
  constraint horizontal L8
  constraint vertical L9
  constraint horizontal L10
  constraint vertical L11
  constraint coincident L4.end L5.start
  constraint horizontal L12
  constraint vertical L13
  constraint horizontal L14
  constraint vertical L15
  constraint coincident L5.end L6.start
  constraint horizontal L16
  constraint vertical L17
  constraint horizontal L18
  constraint vertical L19
  constraint coincident L6.end L7.start
  constraint horizontal L20
  constraint vertical L21
  constraint horizontal L22
  constraint vertical L23
  constraint coincident L4.start L7.end
  constraint collinear L9 L13
  constraint collinear L17 L21
  constraint collinear L10 L22
  constraint collinear L14 L18
  measures "d185" distance of L8.end L9.end
  measures "d186" distance of L4.end L8.end
  measures "d187" distance of L4.start L20.end
  measures "d188" distance of L12.end L13.end
extrude "Extrude14" add sketch "Sketch17" against normal blind 19 from surface at -10 contours L7 L20 L21 L22 L23 | L5 L8 L9 L10 L11 | L7 L16 L17 L18 L19 | L5 L12 L13 L14 L15 bodies 35
fillet "Fillet1'''" radius 5 8 edges at (-36, -42, -3.15) (-36, -52, -3.15) (-36, 83, -3.15) (-36, 93, -3.15) (125, -52, -3.15) (125, -42, -3.15) (125, 83, -3.15) (125, 93, -3.15) on bodies 35
sketch "Sketch18" plane through (0, 0, -12.65) normal (0, 0, 1) x (-1, 0, 0)
  line L0 (-147, 49) -> (-147, 10)
  line L1 (-147, 10) -> (-282, 10)
  line L2 (-282, 10) -> (-282, 49)
  line L3 (-282, 49) -> (-147, 49)
  line L4 (-189.5, -93) -> (-144, -93)
  line L5 (-144, -93) -> (-144, 52)
  line L6 (-144, 52) -> (-285, 52)
  line L7 (-285, 52) -> (-285, -93)
  line L8 (-285, -93) -> (-230, -93)
  line L9 (-230, -93) -> (-230, -86)
  line L10 (-230, -86) -> (-233, -86)
  line L11 (-233, -86) -> (-233, -90)
  line L12 (-233, -90) -> (-282, -90)
  line L13 (-282, -90) -> (-282, 7)
  line L14 (-282, 7) -> (-147, 7)
  line L15 (-147, 7) -> (-147, -90)
  line L16 (-147, -90) -> (-186.5, -90)
  line L17 (-186.5, -90) -> (-186.5, -86)
  line L18 (-186.5, -86) -> (-189.5, -86)
  line L19 (-189.5, -86) -> (-189.5, -93)
  line L20 (-144, -93) -> (-134, -93)
  line L21 (-134, -93) -> (-134, -83)
  line L22 (-134, -83) -> (-144, -83)
  line L23 (-144, -83) -> (-144, -93)
  line L24 (-285, -93) -> (-295, -93)
  line L25 (-295, -93) -> (-295, -83)
  line L26 (-295, -83) -> (-285, -83)
  line L27 (-285, -83) -> (-285, -93)
  line L28 (-144, 52) -> (-134, 52)
  line L29 (-134, 52) -> (-134, 42)
  line L30 (-134, 42) -> (-144, 42)
  line L31 (-144, 42) -> (-144, 52)
  line L32 (-285, 52) -> (-295, 52)
  line L33 (-295, 52) -> (-295, 42)
  line L34 (-295, 42) -> (-285, 42)
  line L35 (-285, 42) -> (-285, 52)
  dimension "d194" = 10
  dimension "d195" = 10
  dimension "d197" = 10
  dimension "d198" = 10
  dimension "d199" = 10
  dimension "d200" = 10
  constraint horizontal L20
  constraint vertical L21
  constraint horizontal L22
  constraint vertical L23
  constraint coincident L4.end L5.start
  constraint horizontal L24
  constraint vertical L25
  constraint horizontal L26
  constraint vertical L27
  constraint coincident L7.end L8.start
  constraint horizontal L28
  constraint vertical L29
  constraint horizontal L30
  constraint vertical L31
  constraint coincident L5.end L6.start
  constraint horizontal L32
  constraint vertical L33
  constraint horizontal L34
  constraint vertical L35
  constraint coincident L6.end L7.start
  constraint collinear L22 L26
  constraint collinear L21 L29
  measures "d194" distance of L33.end L34.end
  measures "d195" distance of L32.end L33.end
  measures "d197" distance of L7.end L24.end
  measures "d198" distance of L28.end L29.end
  measures "d199" distance of L29.end L30.end
  measures "d200" distance of L20.end L21.end
extrude "Extrude15" add sketch "Sketch18" against normal blind 20 contours L5 L20 L21 L22 L23 | L5 L28 L29 L30 L31 | L7 L32 L33 L34 L35 | L7 L24 L25 L26 L27 bodies 34
fillet "Fillet2" radius 5 4 edges at (134, 93, -22.65) (134, -52, -22.65) (295, 93, -22.65) (295, -52, -22.65) on bodies 34
sketch "Sketch19" plane through (0, 0, -32.65) normal (0, 0, -1) x (1, 0, 0)
  arc A0 (134, -88) -> (139, -93) centre (139, -88) ccw
  line L0 (139, -93) -> (290, -93)
  arc A1 (290, -93) -> (295, -88) centre (290, -88) ccw
  line L1 (295, -83) -> (285, -83)
  line L2 (285, -83) -> (285, 42)
  arc A2 (295, 47) -> (290, 52) centre (290, 47) ccw
  line L3 (290, 52) -> (139, 52)
  arc A3 (139, 52) -> (134, 47) centre (139, 47) ccw
  line L4 (134, 42) -> (144, 42)
  line L5 (144, 42) -> (144, -83)
  line L6 (144, -83) -> (134, -83)
  line L7 (134, 47) -> (134, 42)
  line L8 (134, -83) -> (134, -88)
  line L9 (295, -88) -> (295, -83)
  line L10 (295, 42) -> (295, 47)
  line L11 (134, -83) -> (139, -83)
  line L12 (139, -83) -> (139, 42)
  line L13 (139, 42) -> (134, 42)
  line L14 (134, 42) -> (134, -83)
  line L15 (295, -83) -> (290, -83)
  line L16 (290, -83) -> (290, 42)
  line L17 (290, 42) -> (295, 42)
  line L18 (295, 42) -> (295, -83)
  dimension "d205" = 5
  constraint horizontal L11
  constraint vertical L12
  constraint horizontal L13
  constraint vertical L14
  constraint midpoint L4 L12.end
  constraint coincident L6.end L8.start
  constraint horizontal L15
  constraint vertical L16
  constraint horizontal L17
  constraint vertical L18
  constraint coincident L1.start L9.end
  measures "d205" distance of L16 L18
extrude "Extrude16" add sketch "Sketch19" against normal blind 8 contours L4 L6 L11 L12 L13 L14 | L1 L15 L16 L17 L18 bodies 34
sketch "Sketch20" plane through (0, 0, 16.35) normal (0, 0, 1) x (-1, 0, 0)
  line L0 (-98, -83.5) -> (-98, -32.5)
  arc A0 (-93, -27.5) -> (-98, -32.5) centre (-93, -32.5) ccw
  line L1 (-93, -27.5) -> (6, -27.5)
  arc A1 (11, -32.5) -> (6, -27.5) centre (6, -32.5) ccw
  line L2 (11, -32.5) -> (11, -83.5)
  arc A2 (6, -88.5) -> (11, -83.5) centre (6, -83.5) ccw
  line L3 (6, -88.5) -> (-93, -88.5)
  arc A3 (-98, -83.5) -> (-93, -88.5) centre (-93, -83.5) ccw
  line L4 (-115, -93) -> (26, -93)
  line L5 (26, -93) -> (26, 52)
  line L6 (26, 52) -> (-115, 52)
  line L7 (-115, 52) -> (-115, -93)
  line L8 (21, 10) -> (-110, 10)
  line L9 (-110, 10) -> (-110, 52)
  line L10 (-110, 52) -> (21, 52)
  line L11 (21, 52) -> (21, 10)
  line L12 (23, 10) -> (-112, 10)
  line L13 (-112, 10) -> (-112, 52)
  line L14 (-112, 52) -> (23, 52)
  line L15 (23, 52) -> (23, 10)
  dimension "d209" = 5
  dimension "d210" = 5
  dimension "d211" = 42
  dimension "d214" = 2
  dimension "d215" = 2
  constraint horizontal L8
  constraint vertical L9
  constraint horizontal L10
  constraint vertical L11
  constraint coincident L6 L9.end
  constraint horizontal L12
  constraint vertical L13
  constraint horizontal L14
  constraint vertical L15
  constraint coincident L6 L13.end
  constraint collinear L8 L12
  measures "d209" distance of L5 L11
  measures "d210" distance of L7 L9
  measures "d211" distance of L8.end L9.end
  measures "d214" distance of L9 L13
  measures "d215" distance of L11 L15
extrude "Extrude17" cut sketch "Sketch20" against normal blind 3 contours L6 L8 L9 L10 L11 L12 L14 bodies 35
extrude "Extrude18" cut sketch "Sketch20" against normal blind 1.5 contours L6 L9 L12 L13 L14 | L6 L11 L12 L14 L15 bodies 35
sketch "Sketch21" plane through (0, -52, 0) normal (0, -1, 0) x (1, 0, 0)
  line L0 (-23, 14.85) -> (-23, 16.35)
  line L1 (-23, 16.35) -> (-26, 16.35)
  line L2 (-26, 16.35) -> (-26, 6.35)
  line L3 (-26, 6.35) -> (-31, 6.35)
  line L4 (-31, 6.35) -> (-31, -12.65)
  line L5 (-31, -12.65) -> (120, -12.65)
  line L6 (120, -12.65) -> (120, 6.35)
  line L7 (120, 6.35) -> (115, 6.35)
  line L8 (115, 6.35) -> (115, 16.35)
  line L9 (115, 16.35) -> (112, 16.35)
  line L10 (112, 16.35) -> (112, 14.85)
  line L11 (112, 14.85) -> (110, 14.85)
  line L12 (110, 14.85) -> (110, 13.35)
  line L13 (110, 13.35) -> (-21, 13.35)
  line L14 (-21, 13.35) -> (-21, 14.85)
  line L15 (-21, 14.85) -> (-23, 14.85)
  line L16 (-21, 14.85) -> (-23.5, 14.85)
  line L17 (-23.5, 14.85) -> (-23.5, 13.35)
  line L18 (-23.5, 13.35) -> (-21, 13.35)
  line L19 (-21, 13.35) -> (-21, 14.85)
  line L20 (110, 14.85) -> (112.5, 14.85)
  line L21 (112.5, 14.85) -> (112.5, 13.35)
  line L22 (112.5, 13.35) -> (110, 13.35)
  line L23 (110, 13.35) -> (110, 14.85)
  line L24 (42, 14.85) -> (47, 14.85)
  line L25 (47, 14.85) -> (47, 13.35)
  line L26 (47, 13.35) -> (42, 13.35)
  line L27 (42, 13.35) -> (42, 14.85)
  dimension "d218" = 2.5
  dimension "d219" = 1.5
  dimension "d220" = 2.5
  dimension "d221" = 1.5
  dimension "d222" = 5
  dimension "d223" = 63
  constraint horizontal L16
  constraint vertical L17
  constraint horizontal L18
  constraint vertical L19
  constraint coincident L14.end L15.start
  constraint horizontal L20
  constraint vertical L21
  constraint horizontal L22
  constraint vertical L23
  constraint coincident L11.end L12.start
  constraint horizontal L24
  constraint vertical L25
  constraint horizontal L26
  constraint vertical L27
  constraint coincident L13 L25.end
  measures "d218" distance of L14.end L16.end
  measures "d219" distance of L11.end L12.end
  measures "d220" distance of L11.end L20.end
  measures "d221" distance of L24.start L26.end
  measures "d222" distance of L24.start L24.end
  measures "d223" distance of L14.end L24.start
extrude "Extrude19" cut sketch "Sketch21" against normal blind 5 contours L14 L15 L16 L17 L18 L19 | L11 L12 L20 L21 L22 L23 bodies 35
extrude "Extrude20" cut sketch "Sketch21" against normal blind 5 from surface at -42 contours L13 L24 L25 L26 L27 bodies 35
sketch "Sketch22" plane through (0, 0, 16.35) normal (0, 0, 1) x (-1, 0, 0)
  line L0 (19.2606, 78.9381) -> (-115.7394, 78.9381)
  line L1 (-115.7394, 78.9381) -> (-115.7394, 120.9381)
  line L2 (-115.7394, 120.9381) -> (19.2606, 120.9381)
  line L3 (19.2606, 120.9381) -> (19.2606, 78.9381)
  dimension "d229" = 42
  dimension "d230" = 135
  constraint horizontal L0
  constraint vertical L1
  constraint horizontal L2
  constraint vertical L3
  measures "d229" distance of L0.start L2.end
  measures "d230" distance of L0.start L0.end
extrude "Extrude21" add sketch "Sketch22" along normal blind 3 separate body makes body 36
sketch "Sketch23" plane through (0, 0, 19.35) normal (0, 0, 1) x (-1, 0, 0)
  line L0 (19.2606, 120.9381) -> (-115.7394, 120.9381)
  line L1 (-115.7394, 120.9381) -> (-115.7394, 78.9381)
  line L2 (-115.7394, 78.9381) -> (19.2606, 78.9381)
  line L3 (19.2606, 78.9381) -> (19.2606, 120.9381)
  line L4 (19.2606, 78.9381) -> (17.2606, 78.9381)
  line L5 (17.2606, 78.9381) -> (17.2606, 120.9381)
  line L6 (17.2606, 120.9381) -> (19.2606, 120.9381)
  line L7 (19.2606, 120.9381) -> (19.2606, 78.9381)
  line L8 (-115.7394, 78.9381) -> (-113.7394, 78.9381)
  line L9 (-113.7394, 78.9381) -> (-113.7394, 120.9381)
  line L10 (-113.7394, 120.9381) -> (-115.7394, 120.9381)
  line L11 (-115.7394, 120.9381) -> (-115.7394, 78.9381)
  dimension "d233" = 2
  dimension "d234" = 2
  constraint horizontal L4
  constraint vertical L5
  constraint horizontal L6
  constraint vertical L7
  constraint coincident L2.end L3.start
  constraint horizontal L8
  constraint vertical L9
  constraint horizontal L10
  constraint vertical L11
  constraint coincident L1.end L2.start
  measures "d233" distance of L2.end L4.end
  measures "d234" distance of L1.end L8.end
extrude "Extrude22" cut sketch "Sketch23" against normal blind 1.5 contours L0 L2 L3 L4 L5 L6 L7 | L0 L1 L2 L8 L9 L10 L11 bodies 36
move_body "Move17" bodies 36 to x (1, 0, 0) y (0, -1, 0) z (0, 0, -1) at (0, -199.8761, 38.7)
sketch "Sketch24" plane through (0, -78.9381, 0) normal (0, 1, 0) x (-1, 0, 0)
  line L0 (17.2606, 19.35) -> (17.2606, 20.85)
  line L1 (17.2606, 20.85) -> (19.2606, 20.85)
  line L2 (19.2606, 20.85) -> (19.2606, 22.35)
  line L3 (19.2606, 22.35) -> (-115.7394, 22.35)
  line L4 (-115.7394, 22.35) -> (-115.7394, 20.85)
  line L5 (-115.7394, 20.85) -> (-113.7394, 20.85)
  line L6 (-113.7394, 20.85) -> (-113.7394, 19.35)
  line L7 (-113.7394, 19.35) -> (17.2606, 19.35)
  line L8 (-50.7394, 19.35) -> (-45.7394, 19.35)
  line L9 (-45.7394, 19.35) -> (-45.7394, 20.85)
  line L10 (-45.7394, 20.85) -> (-50.7394, 20.85)
  line L11 (-50.7394, 20.85) -> (-50.7394, 19.35)
  dimension "d237" = 5
  dimension "d238" = 1.5
  dimension "d239" = 63
  constraint horizontal L8
  constraint vertical L9
  constraint horizontal L10
  constraint vertical L11
  constraint coincident L7 L8.start
  measures "d237" distance of L9.end L10.end
  measures "d238" distance of L8.end L9.end
  measures "d239" horizontal distance of L5.end L8.start
extrude "Extrude23" add sketch "Sketch24" along normal blind 5 contours L7 L8 L9 L10 L11 bodies 36
sketch "Sketch25" plane through (0, -120.9381, 0) normal (0, -1, 0) x (1, 0, 0)
  line L0 (-17.2606, 20.85) -> (-17.2606, 19.35)
  line L1 (-17.2606, 19.35) -> (113.7394, 19.35)
  line L2 (113.7394, 19.35) -> (113.7394, 20.85)
  line L3 (113.7394, 20.85) -> (115.7394, 20.85)
  line L4 (115.7394, 20.85) -> (115.7394, 22.35)
  line L5 (115.7394, 22.35) -> (-19.2606, 22.35)
  line L6 (-19.2606, 22.35) -> (-19.2606, 20.85)
  line L7 (-19.2606, 20.85) -> (-17.2606, 20.85)
  line L8 (-17.2606, 20.85) -> (-19.7606, 20.85)
  line L9 (-19.7606, 20.85) -> (-19.7606, 19.35)
  line L10 (-19.7606, 19.35) -> (-17.2606, 19.35)
  line L11 (-17.2606, 19.35) -> (-17.2606, 20.85)
  line L12 (113.7394, 20.85) -> (116.2394, 20.85)
  line L13 (116.2394, 20.85) -> (116.2394, 19.35)
  line L14 (116.2394, 19.35) -> (113.7394, 19.35)
  line L15 (113.7394, 19.35) -> (113.7394, 20.85)
  dimension "d242" = 2.5
  dimension "d243" = 2.5
  constraint horizontal L8
  constraint vertical L9
  constraint horizontal L10
  constraint vertical L11
  constraint coincident L0.start L7.end
  constraint horizontal L12
  constraint vertical L13
  constraint horizontal L14
  constraint vertical L15
  constraint coincident L2.end L3.start
  constraint collinear L1 L14
  constraint collinear L1 L10
  measures "d242" distance of L0.start L8.end
  measures "d243" distance of L2.end L12.end
extrude "Extrude24" add sketch "Sketch25" against normal blind 5 contours L0 L7 L8 L9 L10 L11 | L2 L3 L12 L13 L14 L15 bodies 36
move_body "Move18" bodies 36 to x (1, 0, 0) y (0, 1, 0) z (0, 0, 1) at (-4, 0, -5)